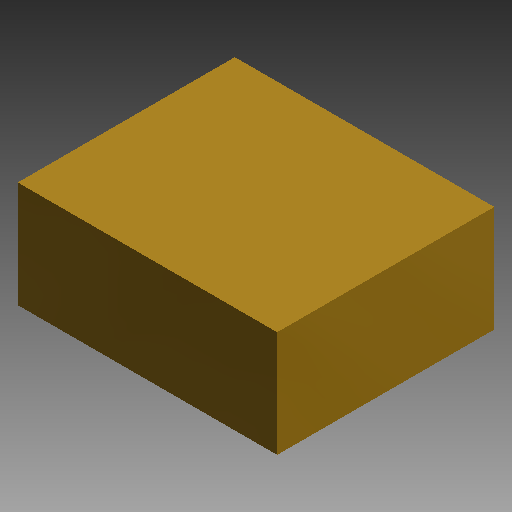
# Autodesk Inventor part: 5x2 IDCw
Saved by Autodesk Inventor 2018.2 (Build 222227000, 227)
## iProperties
Part Number: 5x2 IDCw
Material: Generic
Document SubType Name: Modeling
Designer: autocad
Appearance: 2X5 IDCW, 5x2 IDCw
Author: autocad
Autodesk Inventor part; units mm, degrees
ref_plane "YZ Plane" through (0, 0, 0) normal (1, 0, 0) x (0, 1, 0)
ref_plane "XZ Plane" through (0, 0, 0) normal (0, 1, 0) x (-1, 0, 0)
ref_plane "XY Plane" through (0, 0, 0) normal (0, 0, 1) x (1, 0, 0)
sketch "2X5 IDCW, 5x2 IDCw_11" plane through (0, 0, 0) normal (0, 0, 1) x (1, 0, 0)
  line L0 (11.53, 3.91) -> (11.53, -1.37)
  line L1 (11.53, -1.37) -> (-1.37, -1.37)
  line L2 (-1.37, -1.37) -> (-1.37, 3.91)
  line L3 (-1.37, 3.91) -> (11.53, 3.91)
  constraints: 8 end point
extrude "Extrusion1" add sketch "2X5 IDCW, 5x2 IDCw_11" along normal blind 10.795
body "Solid1"
